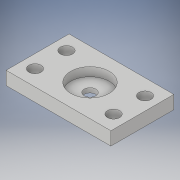
# Autodesk Inventor part: bracket for drone
Saved by Autodesk Inventor 2019.4 (Build 234330000, 330)
## iProperties
Created: 2019-06-13
Part Number: bracket for drone
Material: Generic
Document SubType Name: Modeling
Designer: abdel
Density: 1 g/cm^3
Appearance: Default
Author: abdel
Autodesk Inventor part; units mm, degrees
ref_plane "YZ Plane" through (0, 0, 0) normal (1, 0, 0) x (0, 1, 0)
ref_plane "XZ Plane" through (0, 0, 0) normal (0, 1, 0) x (-1, 0, 0)
ref_plane "XY Plane" through (0, 0, 0) normal (0, 0, 1) x (1, 0, 0)
sketch "Sketch1" plane through (0, 0, 0) normal (0, 1, 0) x (-1, 0, 0)
  circle A0 centre (0, 0) radius 4.2386
  circle A1 centre (0, 0) radius 14.0056
  line L0 (0, 0) -> (0, 22.8956)
  line L1 (0, 0) -> (0, -22.8956)
  line L2 (0, 22.8956) -> (38.1, 22.8956)
  line L3 (0, -22.8956) -> (-38.1, -22.8956)
  line L4 (38.1, 22.8956) -> (-38.1, 22.8956)
  line L5 (-38.1, 22.8956) -> (-38.1, -22.8956)
  line L6 (-38.1, -22.8956) -> (38.1, -22.8956)
  line L7 (38.1, -22.8956) -> (38.1, 22.8956)
  line L8 (19.05, 22.8956) -> (38.1, 22.8956)
  line L9 (38.1, 22.8956) -> (19.05, 22.8956)
  line L10 (19.05, -22.8956) -> (38.1, -22.8956)
  line L11 (38.1, -22.8956) -> (38.1, 22.8956)
  line L12 (38.1, 22.8956) -> (19.05, 22.8956)
  line L13 (19.05, 22.8956) -> (19.05, -22.8956)
  line L14 (38.1, 22.8956) -> (28.575, 22.8956)
  circle A2 centre (28.575, 11.4465) radius 4.445
  circle A3 centre (28.575, -11.4516) radius 4.445
  line L15 (-19.05, -22.8956) -> (-19.05, 22.8956)
  line L16 (-38.1, 22.8956) -> (-19.05, 22.8956)
  line L17 (-19.05, 22.8956) -> (-38.1, 22.8956)
  line L18 (-38.1, -22.8956) -> (-19.05, -22.8956)
  line L19 (-19.05, -22.8956) -> (-19.05, 22.8956)
  line L20 (-19.05, 22.8956) -> (-38.1, 22.8956)
  line L21 (-38.1, 22.8956) -> (-38.1, -22.8956)
  line L22 (-19.05, 22.8956) -> (-28.575, 22.8956)
  circle A4 centre (-28.575, 11.4465) radius 4.445
  circle A5 centre (-28.575, -11.4516) radius 4.445
  dimension "d0" = 8.4772
  dimension "d1" = 28.0111
  dimension "d11" = 22.8956
  dimension "d12" = 22.8956
  dimension "d13" = 38.1
  dimension "d14" = 38.1
  dimension "d15" = 45.7911
  dimension "d16" = 76.2
  dimension "d27" = 45.7911
  dimension "d28" = 19.05
  dimension "d29" = 19.05
  dimension "d30" = 9.525
  dimension "d31" = 8.89
  dimension "d32" = 45.7911
  dimension "d33" = 45.7911
  dimension "d34" = 19.05
  dimension "d35" = 19.05
  dimension "d36" = 9.525
  dimension "d37" = 8.89
  constraints: 46 end point, 7 horizontal, 6 centre point, 4 parallel, 3 perpendicular, 2 coincident, 2 midpoint, 2 vertical
  measures "d0" diameter of A0
  measures "d1" diameter of A1
  measures "d11" distance of L0.start L0.end
  measures "d12" distance of L0.start L1.end
  measures "d13" distance of L0.end L2.end
  measures "d14" distance of L1.end L3.end
  measures "d15" distance of L6.end L2.end
  measures "d16" distance of L3.end L6.end
  measures "d27" distance of L10.end L8.end
  measures "d28" distance of L10.start L10.end
  measures "d29" distance of L8.start L8.end
  measures "d30" distance of L8.end L14.end
  measures "d31" diameter of A2
  measures "d32" distance of L15.start L15.end
  measures "d33" distance of L18.end L19.end
  measures "d34" distance of L21.end L18.end
  measures "d35" distance of L21.start L19.end
  measures "d36" distance of L19.end L22.end
  measures "d37" diameter of A4
sketch "Sketch2" plane through (0, 0, 0) normal (0, 1, 0) x (-1, 0, 0)
  circle A0 centre (0, 0) radius 4.2386
  circle A1 centre (0, 0) radius 14.0056
  line L0 (0, 0) -> (0, 22.8956)
  line L1 (0, 0) -> (0, -22.8956)
  line L2 (0, 22.8956) -> (38.1, 22.8956)
  line L3 (0, -22.8956) -> (-38.1, -22.8956)
  line L4 (38.1, 22.8956) -> (-38.1, 22.8956)
  line L5 (-38.1, 22.8956) -> (-38.1, -22.8956)
  line L6 (-38.1, -22.8956) -> (38.1, -22.8956)
  line L7 (38.1, -22.8956) -> (38.1, 22.8956)
  dimension "d17" = 8.4772
  dimension "d18" = 28.0111
  dimension "d19" = 22.8956
  dimension "d20" = 22.8956
  dimension "d21" = 38.1
  dimension "d22" = 38.1
  dimension "d23" = 45.7911
  dimension "d24" = 76.2
  constraints: 16 end point, 3 horizontal, 2 centre point, 2 coincident, 2 parallel, 2 vertical, 1 perpendicular
  measures "d17" diameter of A0
  measures "d18" diameter of A1
  measures "d19" distance of L0.start L0.end
  measures "d20" distance of L0.start L1.end
  measures "d21" distance of L0.end L2.end
  measures "d22" distance of L1.end L3.end
  measures "d23" distance of L6.end L2.end
  measures "d24" distance of L3.end L6.end
extrude "Extrusion2" add sketch "Sketch2" along normal blind 3.302 contours A0 L0 A1 L1 | A0 L1 A1 L0
extrude "Extrusion3" add sketch "Sketch1" along normal blind 9.652 contours L0 L2 L13 L6 L1 A1 | A1 L1 L3 L15 L4 L0 | L2 L7 L6 L13 | L15 L3 L5 L4
body "Solid1"
